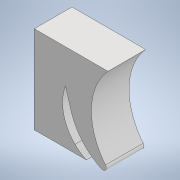
# Autodesk Inventor part: TRIGGER_2
Saved by Autodesk Inventor 2022 (Build 260153000, 153)
## iProperties
Created: 2022-05-17
Part Number: TRIGGER_2
Material: Generic
Document SubType Name: Sheet Metal
Designer: joshn
Density: 1 g/cm^3
Sheet Metal Rule: Default
Appearance: Default
Author: joshn
Autodesk Inventor part; units mm, degrees
ref_plane "YZ Plane" through (0, 0, 0) normal (1, 0, 0) x (0, 1, 0)
ref_plane "XZ Plane" through (0, 0, 0) normal (0, 1, 0) x (-1, 0, 0)
ref_plane "XY Plane" through (0, 0, 0) normal (0, 0, 1) x (1, 0, 0)
sketch "Sketch1" plane through (0, 0, 0) normal (1, 0, 0) x (0, 1, 0)
  point P0 (0, 0)
sketch "Sketch2" plane through (0, 0, 0) normal (0, 0, 1) x (1, 0, 0)
  line L0 (4.0785, 4.9113) -> (2.4908, 4.9113) construction
  line L1 (4.0785, 3.7037) -> (4.0785, 4.9113) construction
  line L2 (2.4323, 3.7037) -> (4.0785, 3.7037) construction
  arc A0 (2.4323, 3.7037) -> (2.2344, -2.9627) centre (6.1869, 0.2561) ccw
  arc A1 (1.8925, -3.3998) -> (2.2344, -2.9627) centre (2.0138, -3.1424) ccw
  arc A2 (-0.5696, -0.5268) -> (1.8925, -3.3998) centre (3.8604, 0.7782) ccw
  line L3 (-1.0058, 0.9542) -> (-0.5696, -0.5268)
  arc A3 (-1.0058, 0.9542) -> (-0.2339, -2.7516) centre (2.2087, -0.3095) ccw
  arc A4 (-0.2339, -2.7516) -> (1.9052, -3.655) centre (1.9474, -0.5708) ccw
  line L4 (2.5244, -3.655) -> (1.9052, -3.655) construction
  line L5 (2.5244, -4.0286) -> (2.5244, -3.655) construction
  line L6 (1.9895, -4.0228) -> (2.5244, -4.0286) construction
  line L7 (1.9895, -3.8389) -> (1.9895, -4.0228) construction
  line L8 (1.9474, -3.8389) -> (1.9895, -3.8389) construction
  arc A5 (0.288, -3.3863) -> (1.9474, -3.8389) centre (1.9474, -0.5708) ccw construction
  line L9 (-3.5298, -3.3863) -> (0.288, -3.3863) construction
  line L10 (-3.5298, 3.7037) -> (-3.5298, -3.3863) construction
  line L11 (1.3533, 3.7037) -> (-3.5298, 3.7037) construction
  line L12 (2.4908, 4.9113) -> (1.3533, 3.7037) construction
  line L13 (0.288, -3.3863) -> (0.6877, -3.3863)
  line L14 (2.4323, 3.7037) -> (-3.5298, 3.7037)
  line L15 (-3.5298, -3.3863) -> (-3.5298, 3.7037)
  line L16 (0.288, -3.3863) -> (-3.5298, -3.3863)
  point P0 (0, 0)
extrude "Plate1" add sketch "Sketch2" along normal blind 3.048
equation "\"d0\" = Thickness"
equation "\"BendRadius\" = Thickness"
equation "\"BendReliefWidth\" = Thickness"
equation "\"BendReliefDepth\" = 0.5 * Thickness"
equation "\"CornerReliefSize\" = 4 * Thickness"
equation "\"MinimumRemnant\" = 2 * Thickness"
equation "\"TransitionRadius\" = BendRadius"
equation "\"JacobiRadiusSize\" = BendRadius"
equation "\"GapSize\" = Thickness"
equation "\"Thickness\" = 3.048"
body "Solid1"
